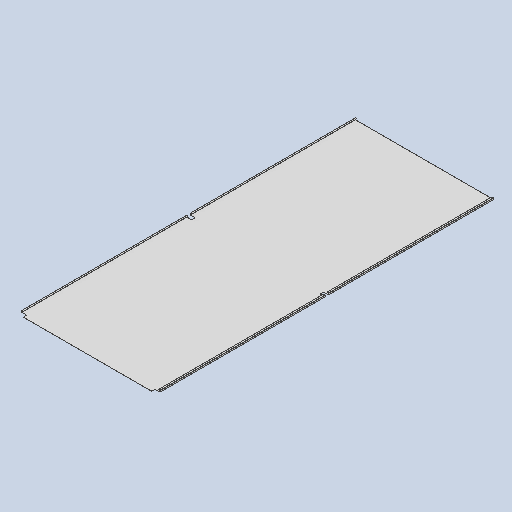
# Autodesk Inventor part: MSC 804 sheet gills
Saved by Autodesk Inventor 2025 (Build 290162010, 162A)
## iProperties
Created: 2024-06-15
Part Number: MSC 804 sheet gills
Material: Stainless Steel
Document SubType Name: Sheet Metal
Designer: pokla
Stock Number: МОО 804 лист жабра
Mass: 6723.7 g
Surface Area: 33647.6 cm^2
Volume: 840.462 cm^3
Density: 8 g/cm^3
Sheet Metal Rule: Default_mm
Appearance: Default
Flat Pattern Width: 85.0724 cm
Flat Pattern Length: 198 cm
Flat Pattern Area: 16844.3 cm^2
Sheet Metal Width: 850,724 mm
Sheet Metal Length: 1980,000 mm
Sheet Metal Area: 1684433,309 mm^2
Author: pokla
Autodesk Inventor part; units mm, degrees
ref_plane "YZ Plane" through (0, 0, 0) normal (1, 0, 0) x (0, 1, 0)
ref_plane "XZ Plane" through (0, 0, 0) normal (0, 1, 0) x (-1, 0, 0)
ref_plane "XY Plane" through (0, 0, 0) normal (0, 0, 1) x (1, 0, 0)
sketch "Sketch6" plane through (0, 0, 0) normal (0, 1, 0) x (-1, 0, 0)
  line L0 (407.1, -990) -> (-407.1, -990)
  line L1 (-407.1, -990) -> (-407.1, 990)
  line L2 (-407.1, 990) -> (407.1, 990)
  line L3 (407.1, 990) -> (407.1, -990)
  line L4 (407.1, -990) -> (-407.1, 990) construction
  line L5 (-407.1, -990) -> (407.1, 990) construction
  point P0 (0, 0)
  dimension "d52" = 814.2
  dimension "d53" = 1980
  measures "d52" distance of L1.end L2.end
  measures "d53" distance of L0.end L1.end
extrude "Plate2" add sketch "Sketch6" along normal blind 0.5
sketch "Sketch10" plane through (-406.6, 0, 990) normal (-1, 0, 0) x (0, -1, 0)
  line L0 (0, -1980) -> (0, 0)
  line L1 (0, 0) -> (-10, 0)
  line L2 (-10, 0) -> (-10, -1980)
  line L3 (-10, -1980) -> (0, -1980)
  constraints: 6 end point, 1 horizontal, 1 perpendicular, 1 vertical
edge flange "Flange1" height 10 angle 90 thickness 0.5 bend radius 0.5 thickness toward (-1, 0, 0) relief straight relief width 0.5 relief depth 0.25 corner gap 0.5 corner form 0 edges at (-407.1, 0.5, 0) (407.1, 0.5, 0) wall of the first edge with corners at (-406.6, 0, -990) (-406.6, 0, 990) (-406.6, 10, 990) (-406.6, 10, -990)
bend "Bend2"
corner "Corner2"
sketch "Sketch11" plane through (407.1, 9.5, -990) normal (0, 1, 0) x (-1, 0, 0)
  line L0 (0, 1980) -> (0, 0)
  line L1 (0, 0) -> (10, 0)
  line L2 (10, 0) -> (10, 1980)
  line L3 (10, 1980) -> (0, 1980)
  constraints: 6 end point, 1 horizontal, 1 perpendicular, 1 vertical
edge flange "Flange2" height 10 angle 90 thickness 0.5 bend radius 0.5 thickness toward (0, 1, 0) relief straight relief width 0.5 relief depth 0.25 corner gap 0.5 corner form 0 edges at (406.6, 10, 0) (-406.6, 10, 0) wall of the first edge with corners at (407.1, 9.5, 990) (407.1, 9.5, -990) (397.1, 9.5, -990) (397.1, 9.5, 990)
bend "Bend3"
corner "Corner3"
sketch "Sketch12" plane through (0, 0, 0) normal (0, -1, 0) x (1, 0, 0)
  line L0 (-407.1, 990) -> (-377.1, 990)
  line L1 (-377.1, 990) -> (-377.1, 970)
  line L2 (-377.1, 970) -> (-407.1, 970)
  line L3 (-407.1, 970) -> (-407.1, 990)
  line L4 (-407.1, 0) -> (-377.1, 0)
  line L5 (-377.1, 0) -> (-377.1, -20)
  line L6 (-377.1, -20) -> (-407.1, -20)
  line L7 (-407.1, -20) -> (-407.1, 0)
  line L8 (407.1, 0) -> (377.1, 0)
  line L9 (377.1, 0) -> (377.1, -20)
  line L10 (377.1, -20) -> (407.1, -20)
  line L11 (407.1, -20) -> (407.1, 0)
  line L12 (407.1, 990) -> (377.1, 990)
  line L13 (377.1, 990) -> (377.1, 970)
  line L14 (377.1, 970) -> (407.1, 970)
  line L15 (407.1, 970) -> (407.1, 990)
  line L16 (-407.1, -990) -> (-407.1, 990) construction
  line L17 (-406.1, 990) -> (406.1, 990) construction
  line L18 (407.1, 990) -> (407.1, -990) construction
  point P0 (0, 0)
  dimension "d94" = 20
  dimension "d95" = 30
  dimension "d96" = 990
  dimension "d97" = 30
  constraints: 32 end point, 9 collinear, 8 parallel, 4 horizontal, 4 perpendicular, 3 equal length
  measures "d94" distance of L0.end L2.start
  measures "d95" distance of L0.start L0.end
  measures "d96" distance between parallel lines of L4 L0
  measures "d97" distance of L14.start L14.end
extrude "Extrusion3" cut sketch "Sketch12" along normal through all both and the other way through all
fillet "Corner Round1" radius 4 16 edges at (377.1, 0.25, -20) (397.1, 9.75, 970) (377.1, 0.25, 970) (377.1, 0.25, 990) (397.1, 9.75, -20) (377.1, 0.25, 0) (397.1, 9.75, 0) (397.1, 9.75, -990) (-397.1, 9.75, -990) (-397.1, 9.75, -20) (-397.1, 9.75, 0) (-377.1, 0.25, -20) (-377.1, 0.25, 0) (-397.1, 9.75, 970) (-377.1, 0.25, 970) (-377.1, 0.25, 990)
equation "\"d52\" = ЖАБРЫ_базовая_ширина - ЖАБРЫ_шаг_листов"
equation "\"d53\" = ЖАБРЫ_базовая_длина_дл_лист"
equation "\"d97\" = d95"
equation "\"d54\" = Thickness"
equation "\"d74\" = BendReliefWidth"
equation "\"d75\" = BendReliefDepth"
equation "\"d76\" = MinimumRemnant"
equation "\"d77\" = TransitionRadius"
equation "\"d80\" = BendRadius"
equation "\"d81\" = CornerReliefSize"
equation "\"d82\" = GapSize"
equation "\"d83\" = JacobiRadiusSize"
equation "\"d84\" = BendReliefWidth"
equation "\"d85\" = BendReliefDepth"
equation "\"d86\" = MinimumRemnant"
equation "\"d87\" = TransitionRadius"
equation "\"d90\" = BendRadius"
equation "\"d91\" = CornerReliefSize"
equation "\"d92\" = GapSize"
equation "\"d93\" = JacobiRadiusSize"
equation "\"BendRadius\" = Thickness"
equation "\"BendReliefWidth\" = Thickness"
equation "\"BendReliefDepth\" = 0.5 * Thickness"
equation "\"CornerReliefSize\" = 4 * Thickness"
equation "\"MinimumRemnant\" = 2 * Thickness"
equation "\"TransitionRadius\" = BendRadius"
equation "\"JacobiRadiusSize\" = BendRadius"
equation "\"GapSize\" = Thickness"
equation "\"ЖАБРЫ_базовая_ширина\" = 915"
equation "\"ЖАБРЫ_шаг_листов\" = 100.8"
equation "\"ЖАБРЫ_базовая_длина_дл_лист\" = 1980"
equation "\"Thickness\" = 0.5"
body "Solid2"
